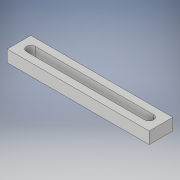
# Autodesk Inventor part: CameraSlider
Saved by Autodesk Inventor 2019 (Build 230136000, 136)
## iProperties
Created: 2019-07-15
Part Number: CameraSlider
Material: Generic
Document SubType Name: Modeling
Designer: aorfi
Density: 1 g/cm^3
Appearance: Default
Author: aorfi
Autodesk Inventor part; units mm, degrees
ref_plane "YZ Plane" through (0, 0, 0) normal (1, 0, 0) x (0, 1, 0)
ref_plane "XZ Plane" through (0, 0, 0) normal (0, 1, 0) x (-1, 0, 0)
ref_plane "XY Plane" through (0, 0, 0) normal (0, 0, 1) x (1, 0, 0)
sketch "Sketch1" plane through (0, 0, 0) normal (0, 1, 0) x (-1, 0, 0)
  line L0 (-30, 5) -> (30, 5)
  line L1 (30, 5) -> (30, -5)
  line L2 (30, -5) -> (-30, -5)
  line L3 (-30, -5) -> (-30, 5)
  line L4 (-30, 5) -> (30, -5) construction
  line L5 (30, 5) -> (-30, -5) construction
  circle A0 centre (25, 0) radius 1.8986
  circle A1 centre (-25, 0) radius 1.8986
  line L6 (25, 1.8987) -> (-25, 1.8987)
  line L7 (-25, -1.8986) -> (25, -1.8986)
  point P0 (0, 0)
  point P1 (0, 0)
  dimension "d0" = 60
  dimension "d1" = 10
  dimension "d2" = 3.7973
  dimension "d3" = 3.7973
  dimension "d4" = 5
  dimension "d5" = 5
  constraints: 16 end point, 4 point on circle, 4 tangent, 3 midpoint, 2 centre point, 2 horizontal, 2 parallel, 1 horizontal alignment, 1 perpendicular
  measures "d0" distance of L1.end L2.end
  measures "d1" distance of L0.end L1.end
  measures "d2" diameter of A0
  measures "d3" diameter of A1
  measures "d4" distance from line of A0.centre L1
  measures "d5" distance from line of L3 A1.centre
extrude "Extrusion1" add sketch "Sketch1" along normal mid plane 5
equation "\"d3\" = d2"
equation "\"d5\" = d4"
body "Solid1"
